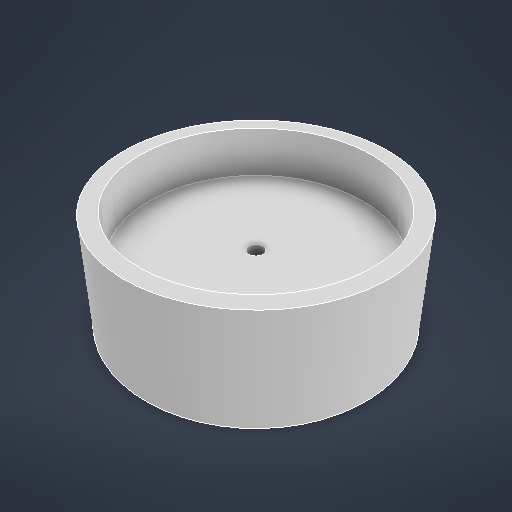
# Autodesk Inventor part: Wheel
Saved by Autodesk Inventor 2025 (Build 290162000, 162)
## iProperties
Created: 2024-05-20
Part Number: Wheel
Material: Generic
Document SubType Name: Modeling
Designer: Garfieldcmix
Density: 1 g/cm^3
Appearance: Default
Author: Garfieldcmix
Autodesk Inventor part; units mm, degrees
ref_plane "YZ Plane" through (0, 0, 0) normal (1, 0, 0) x (0, 1, 0)
ref_plane "XZ Plane" through (0, 0, 0) normal (0, 1, 0) x (-1, 0, 0)
ref_plane "XY Plane" through (0, 0, 0) normal (0, 0, 1) x (1, 0, 0)
sketch "Sketch1" plane through (0, 0, 0) normal (0, 1, 0) x (-1, 0, 0)
  circle A0 centre (0, 0) radius 34
  dimension "d0" = 68
  constraints: 1 centre point, 1 coincident
  measures "d0" diameter of A0
extrude "Extrusion1" add sketch "Sketch1" along normal blind 27
sketch "Sketch2" plane through (0, 27, 0) normal (0, 1, 0) x (1, 0, 0)
  circle A0 centre (0, 0) radius 30
  dimension "d3" = 60
  constraints: 1 centre point, 1 coincident
  measures "d3" diameter of A0
extrude "Extrusion2" cut sketch "Sketch2" against normal blind 12
sketch "Sketch5" plane through (0, 15, 0) normal (0, 1, 0) x (1, 0, 0)
  circle A0 centre (0, 0) radius 2
  dimension "d13" = 4
  constraints: 1 centre point, 1 coincident
  measures "d13" diameter of A0
extrude "Extrusion5" cut sketch "Sketch5" against normal through all
body "Solid1"
